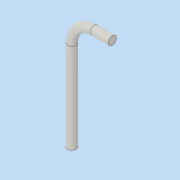
# Autodesk Inventor part: 3mmControlSurfaceShaft_2
Saved by Autodesk Inventor 2017 (Build 210142000, 142)
## iProperties
Created: 2016-10-13
Part Number: 3mmControlSurfaceShaft_2
Material: Generic
Document SubType Name: Modeling
Designer: techn
Density: 1 g/cm^3
Appearance: Steel
Author: techn
Autodesk Inventor part; units mm, degrees
ref_plane "YZ Plane" through (0, 0, 0) normal (1, 0, 0) x (0, 1, 0)
ref_plane "XZ Plane" through (0, 0, 0) normal (0, 1, 0) x (-1, 0, 0)
ref_plane "XY Plane" through (0, 0, 0) normal (0, 0, 1) x (1, 0, 0)
sketch "Sketch1" plane through (0, 0, 0) normal (0, 0, 1) x (1, 0, 0)
  line L0 (0, 0) -> (0, 31.75)
  line L1 (0, 31.75) -> (7.9375, 31.75)
  line L2 (7.9375, 31.75) -> (7.9375, 39.6875)
  line L3 (7.9375, 39.6875) -> (14.2875, 39.6875)
  arc A0 (7.9375, 39.6875) -> (0, 31.75) centre (7.9375, 31.75) ccw
  dimension "d0" = 31.75
  dimension "d1" = 7.9375
  dimension "d2" = 7.9375
  dimension "d3" = 6.35
  constraints: 8 end point, 3 perpendicular, 2 point on circle, 1 centre point, 1 tangent, 1 vertical
  measures "d0" distance of L0.start L0.end
  measures "d1" distance of L0.end L1.end
  measures "d2" distance of L1.end L2.end
  measures "d3" distance of L2.end L3.end
sketch "Sketch2" plane through (0, 0, 0) normal (0, 1, 0) x (-1, 0, 0)
  circle A0 centre (0, 0) radius 1.5
  dimension "d4" = 3
  constraints: 1 centre point, 1 coincident
  measures "d4" diameter of A0
sweep "Sweep1" add profiles "Sketch2" path "Sketch1" path curves L0 A0 L3
body "Solid1"
